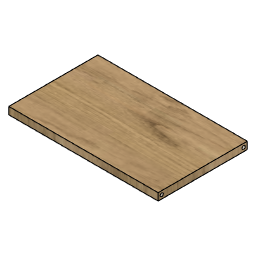
Project 02 (Autodesk Fusion 360 archive; units mm, degrees)
design "Base"
Autodesk Fusion 360 part; units mm, degrees
note: some values were not read from the file. Set by a fixed rule: which face or edge a step refers to.
sketch "Sketch1" plane through (0, 0, 0) normal (0, 1, 0) x (1, 0, 0)
  line L0 (0, 0) -> (310, 0)
  line L1 (310, 0) -> (310, -185)
  line L2 (310, -185) -> (0, -185)
  line L3 (0, -185) -> (0, 0)
  dimension "d1" = 310
  dimension "d2" = 185
  constraint horizontal L0
  constraint vertical L1
  constraint horizontal L2
  constraint vertical L3
  constraint coincident L0.start L3.end
  measures "d1" distance of L0.start L0.end
  measures "d2" distance of L0.start L2.end
extrude "Extrude1" add sketch "Sketch1" along normal blind 15
sketch "Sketch2" plane through (310, 0, 0) normal (1, 0, 0) x (0, 0, -1)
  line L0 (-185, 0) -> (0, 0)
  line L1 (0, 0) -> (0, 15)
  line L2 (0, 15) -> (-185, 15)
  line L3 (-185, 15) -> (-185, 0)
  circle A0 centre (-177.5, 7.5) radius 4
  circle A1 centre (-7.5, 7.5) radius 4
  line L4 (0, 0) -> (0, 7.5)
  constraint midpoint L1 L4.end
  constraint coincident L0.end L1.start
sketch "Sketch3" plane through (0, 0, 0) normal (-1, 0, 0) x (0, 0, 1)
  line L0 (0, 0) -> (185, 0)
  line L1 (185, 0) -> (185, 15)
  line L2 (185, 15) -> (0, 15)
  line L3 (0, 15) -> (0, 0)
  circle A0 centre (7.5, 7.5) radius 4
  dimension "d11" = 8
  measures "d11" diameter of A0
sketch "Sketch4" plane through (0, 0, 0) normal (-1, 0, 0) x (0, 0, 1)
  circle A0 centre (177.5, 7.5) radius 4
  line L0 (0, 0) -> (7.5, 0) construction
  line L1 (7.5, 0) -> (7.5, 7.5) construction
  line L2 (7.5, 7.5) -> (0, 7.5) construction
  line L3 (0, 7.5) -> (0, 0) construction
  circle A1 centre (7.5, 7.5) radius 4
  dimension "d75" = 7.5
  dimension "d76" = 7.5
  dimension "d77" = 8
  constraint horizontal L0
  constraint vertical L1
  constraint horizontal L2
  constraint vertical L3
  constraint coincident L0.start L3.end
  constraint coincident L1.end L2.start
  measures "d75" distance of L0.start L0.end
  measures "d76" distance of L0.start L2.end
  measures "d77" diameter of A1
extrude "Extrude2" cut sketch "Sketch2" against normal blind 3 contours A0 | A1
thread "Thread1" "ISO Metric profile 8.0 M8x1.25 6H" major diameter 8.17 minor diameter 6.7795 pitch 1.25 angle 60 resizes the face on face at (308, 7.3006, 3.505)
thread "Thread2" "ISO Metric profile 8.0 M8x1.25 6H" major diameter 8.17 minor diameter 6.7795 pitch 1.25 angle 60 resizes the face on face at (308, 10.3635, 180.2929)
sketch "Sketch5" plane through (0, 0, 0) normal (0, 0, -1) x (-1, 0, 0)
  line L0 (-310, 0) -> (0, 0)
  line L1 (0, 0) -> (0, 15)
  line L2 (0, 15) -> (-310, 15)
  line L3 (-310, 15) -> (-310, 0)
  circle A0 centre (-260, 7.5) radius 4
  line L4 (0, 7.5) -> (-50, 7.5)
  circle A1 centre (-50, 7.5) radius 4
  dimension "d21" = 50
  dimension "d22" = 8
  constraint midpoint L1 L4.start
  constraint perpendicular L1 L4
  constraint coincident L4.end A1.centre
  measures "d21" distance of L4.start L4.end
  measures "d22" diameter of A1
sketch "Sketch6" plane through (310, 0, 0) normal (1, 0, 0) x (0, 0, -1)
  circle A0 centre (-177.5, 7.5) radius 3.3898
  line L0 (-185, 0) -> (0, 0)
  line L1 (0, 0) -> (0, 15)
  line L2 (0, 15) -> (-185, 15)
  line L3 (-185, 15) -> (-185, 0)
  circle A1 centre (-7.5, 7.5) radius 4
  circle A2 centre (-7.5, 7.5) radius 3.3898
  dimension "d46" = 8
  measures "d46" diameter of A1
sketch "Sketch7" plane through (0, 0, 0) normal (0, 0, -1) x (-1, 0, 0)
  line L0 (-310, 0) -> (0, 0)
  line L1 (0, 0) -> (0, 15)
  line L2 (0, 15) -> (-310, 15)
  line L3 (-310, 15) -> (-310, 0)
  circle A0 centre (-260, 7.5) radius 4
  dimension "d48" = 8
  dimension "d52" = 0
  measures "d48" diameter of A0
extrude "Extrude16" cut sketch "Sketch7" against normal blind 30 contours A0
thread "Thread11" "ISO Metric profile 8.0 M8x1.25 6H" major diameter 8.17 minor diameter 6.7795 pitch 1.25 angle 60 resizes the face on face at (262.6467, 4.5009, 20)
delete_face "DeleteFace2" 1 faces at (258.4536, 10.5164, 20)
hole "Hole1" at (310, 7.5, 177.5) direction (-1, 0, 0) diameter 6.78 depth 30 tip angle 120
thread "Thread12" "ISO Metric profile 8.0 M8x1.25 6H"
hole "Hole2" at (310, 7.5, 7.5) direction (-1, 0, 0) diameter 6.78 depth 30 tip angle 120
thread "Thread13" "ISO Metric profile 8.0 M8x1.25 6H"
hole "Hole3" at (260, 7.5, 0) direction (0, 0, 1) diameter 6.78 depth 30 tip angle 120
thread "Thread14" "ISO Metric profile 8.0 M8x1.25 6H"
hole "Hole4" at (50, 7.5, 0) direction (0, 0, 1) diameter 6.78 depth 30 tip angle 120
thread "Thread15" "ISO Metric profile 8.0 M8x1.25 6H"
hole "Hole5" at (0, 7.5, 177.5) at (0, 7.5, 7.5) direction (1, 0, 0) diameter 6.78 depth 30 tip angle 120
thread "Thread16" "ISO Metric profile 8.0 M8x1.25 6H"

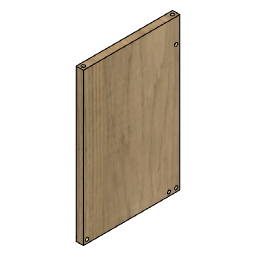
design "Left side"
Autodesk Fusion 360 part; units mm, degrees
sketch "Sketch1" plane through (0, 0, 0) normal (0, 1, 0) x (1, 0, 0)
  line L0 (0, 0) -> (15, 0)
  line L1 (15, 0) -> (15, -200)
  line L2 (15, -200) -> (0, -200)
  line L3 (0, -200) -> (0, 0)
  line L4 (325, -200) -> (340, -200)
  line L5 (340, -200) -> (340, 0)
  line L6 (340, 0) -> (325, 0)
  line L7 (325, 0) -> (325, -200)
  dimension "d1" = 15
  dimension "d2" = 200
  dimension "d3" = 310
  dimension "d4" = 15
  dimension "d5" = 200
  constraint horizontal L0
  constraint vertical L1
  constraint horizontal L2
  constraint vertical L3
  constraint coincident L0.start L3.end
  constraint horizontal L4
  constraint vertical L5
  constraint horizontal L6
  constraint vertical L7
  measures "d1" distance of L0.start L0.end
  measures "d2" distance of L0.start L2.end
  measures "d3" distance of L1.end L4.start
  measures "d4" distance of L4.start L4.end
  measures "d5" distance of L4.start L6.end
sketch "Sketch2" plane through (0, 0, 0) normal (0, 1, 0) x (1, 0, 0)
  line L0 (0, 0) -> (15, 0)
  line L1 (15, 0) -> (15, -200)
  line L2 (15, -200) -> (0, -200)
  line L3 (0, -200) -> (0, 0)
  dimension "d8" = 15
  dimension "d9" = 200
  constraint horizontal L0
  constraint vertical L1
  constraint horizontal L2
  constraint vertical L3
  constraint coincident L0.start L3.end
  measures "d8" distance of L0.start L0.end
  measures "d9" distance of L0.start L2.end
extrude "Extrude2" add sketch "Sketch2" along normal blind 315
sketch "Sketch3" plane through (0, 0, 0) normal (-1, 0, 0) x (0, 0, 1)
  line L0 (0, 0) -> (200, 0)
  line L1 (200, 0) -> (200, 315)
  line L2 (200, 315) -> (0, 315)
  line L3 (0, 315) -> (0, 0)
  circle A0 centre (7.5, 7.5) radius 4
  circle A1 centre (22.5, 7.5) radius 4
  circle A2 centre (192.5, 7.5) radius 4
  circle A3 centre (7.5, 265) radius 4
  dimension "d18" = 8
  dimension "d19" = 8
  dimension "d22" = 8
  dimension "d25" = 8
  measures "d18" diameter of A0
  measures "d19" diameter of A1
  measures "d22" diameter of A2
  measures "d25" diameter of A3
hole "Hole1" at (0, 7.5, 7.5) at (0, 7.5, 22.5) at (0, 265, 7.5) at (0, 7.5, 192.5) direction (1, 0, 0) diameter 6.78 depth 100 tip angle 120 countersink diameter 14.07 countersink angle 90
thread "Thread1" "ISO Metric profile 8.0 M8x1.25 6H"
sketch "Sketch4" plane through (0, 315, 0) normal (0, 1, 0) x (-1, 0, 0)
  line L0 (0, 200) -> (-15, 200)
  line L1 (-15, 200) -> (-15, 0)
  line L2 (-15, 0) -> (0, 0)
  line L3 (0, 0) -> (0, 200)
  circle A0 centre (-7.5, 192.5) radius 4
  circle A1 centre (-7.5, 7.5) radius 4
  dimension "d33" = 8
  dimension "d36" = 8
  measures "d33" diameter of A0
  measures "d36" diameter of A1
hole "Hole2" at (7.5, 315, 192.5) at (7.5, 315, 7.5) direction (0, -1, 0) diameter 6.78 depth 30 tip angle 120
thread "Thread2" "ISO Metric profile 8.0 M8x1.25 6H"

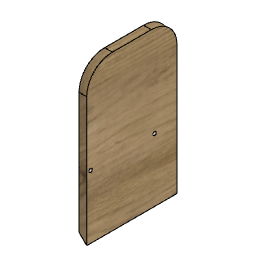
design "T-shape01"
Autodesk Fusion 360 part; units mm, degrees
sketch "Sketch1" plane through (0, 0, 0) normal (0, 1, 0) x (1, 0, 0)
  line L0 (0, 0) -> (21.213, 0)
  line L1 (0, -21.213) -> (0, -21.23)
  line L2 (-201.525, -201.525) -> (0, 0)
  line L3 (21.213, 0) -> (-190.919, -212.132)
  line L4 (-201.525, -201.525) -> (-190.919, -212.132)
  dimension "d1" = 21.213
  dimension "d2" = 21.23
  dimension "d5" = 300
  constraint coincident L0.start L2.end
  constraint horizontal L0
  constraint perpendicular L0 L1
  constraint parallel L2 L3
  constraint coincident L3 L1.start
  measures "d1" distance of L0.start L0.end
  measures "d2" distance of L0.start L1.end
  measures "d5" distance of L0.end L3.end
extrude "Extrude1" add sketch "Sketch1" along normal blind 175
sketch "Sketch2" plane through (10.6065, 0, 10.6065) normal (0.707107, 0, 0.707107) x (0, 1, 0)
  line L0 (0, 285.0001) -> (0, -14.9999)
  line L1 (0, -14.9999) -> (175, -14.9999)
  line L2 (175, -14.9999) -> (175, 285.0001)
  line L3 (175, 285.0001) -> (0, 285.0001)
  arc A0 (50, 285.0001) -> (0, 235.0001) centre (50, 235.0001) ccw
  arc A1 (175, 235.0001) -> (125, 285.0001) centre (125, 235.0001) ccw
  dimension "d8" = 250
  dimension "d9" = 50
  constraint coincident L3 A0.start
  measures "d8" distance of L0.end A0.end
  measures "d9" distance of A0.end A0.centre
extrude "Extrude2" cut sketch "Sketch2" against normal blind 60 contours L0 L3 A0
extrude "Extrude3" cut sketch "Sketch2" against normal blind 90 contours L2 L3 A1
sketch "Sketch3" plane through (0, 0, 0) normal (-0.707107, 0, -0.707107) x (0, -1, 0)
  arc A0 (-125.2749, 284.9994) -> (-175, 235.0001) centre (-125, 235.0001) ccw
  line L0 (-175, 235.0001) -> (-175, 0)
  line L1 (-175, 0) -> (0, 0)
  line L2 (0, 0) -> (0, 235.0001)
  arc A1 (0, 235.0001) -> (-49.7251, 284.9994) centre (-50, 235.0001) ccw
  line L3 (-49.7251, 284.9994) -> (-125.2749, 284.9994)
  line L4 (0, 0) -> (0, 107.5)
  line L5 (-175, 0) -> (-175, 107.5)
  line L6 (-175, 107.5) -> (-131.5, 107.5)
  line L7 (0, 107.5) -> (-7.5, 107.5)
  dimension "d15" = 107.5
  dimension "d16" = 107.5
  dimension "d17" = 43.5
  dimension "d18" = 7.5
  constraint coincident L1.end L2.start
  constraint perpendicular L1 L4
  constraint coincident L0.end L1.start
  constraint perpendicular L1 L5
  constraint perpendicular L0 L6
  constraint perpendicular L4 L7
  measures "d15" distance of L1.end L4.end
  measures "d16" distance of L0.end L5.end
  measures "d17" distance of L5.end L6.end
  measures "d18" distance of L4.end L7.end
hole "Hole1" at (-76.014, 131.5, 76.014) direction (0.707107, 0, 0.707107) diameter 6.78 depth 40 tip angle 120 countersink diameter 14.07 countersink angle 90
thread "Thread4" "ISO Metric profile 8.0 M8x1.25 6H"
thread "Thread1" "ISO Metric profile 8.0 M8x1.25 6H" major diameter 8.17 minor diameter 6.7795 pitch 1.25 angle 60 resizes the face on face at (-73.1387, 131.9215, 83.6462)
hole "Hole2" at (-76.014, 7.5, 76.014) direction (0.707107, 0, 0.707107) diameter 6.78 depth 40 tip angle 120 countersink diameter 14.07 countersink angle 90
thread "Thread3" "ISO Metric profile 8.0 M8x1.25 6H"
thread "Thread2" "ISO Metric profile 8.0 M8x1.25 6H" major diameter 8.17 minor diameter 6.7795 pitch 1.25 angle 60 resizes the face on face at (-67.9644, 10.8858, 83.8246)
sketch "Sketch4" plane through (0, 175, 0) normal (0, 1, 0) x (-1, 0, 0)
  line L0 (166.1702, 166.1702) -> (155.5637, 176.7767)
  line L1 (155.5637, 176.7767) -> (-21.213, 0)
  line L2 (-21.213, 0) -> (0, 0)
  line L3 (0, 0) -> (166.1702, 166.1702)
  circle A0 centre (17.6778, 28.2843) radius 4
  circle A1 centre (70.7108, 81.3173) radius 4
  circle A2 centre (113.1372, 123.7437) radius 4
  dimension "d26" = 75
  dimension "d27" = 60
  dimension "d28" = 8
  dimension "d29" = 8
  dimension "d30" = 8
  measures "d26" distance of A0.centre A1.centre
  measures "d27" distance of A1.centre A2.centre
  measures "d28" diameter of A0
  measures "d29" diameter of A1
  measures "d30" diameter of A2
hole "Hole3" at (-17.6778, 175, 28.2843) at (-70.7108, 175, 81.3173) at (-113.1372, 175, 123.7437) direction (0, -1, 0) diameter 6.78 depth 30 tip angle 120
thread "Thread5" "ISO Metric profile 8.0 M8x1.25 6H"
sketch "Sketch5" plane through (0, 0, 0) normal (0, 0, -1) x (1, 0, 0)
  line L0 (21.213, 0) -> (0, 0)
  line L1 (0, 0) -> (0, -175)
  line L2 (0, -175) -> (21.213, -175)
  line L3 (21.213, -175) -> (21.213, 0)
  circle A0 centre (10.6065, -24.08) radius 4
  circle A1 centre (10.6065, -170) radius 4
  dimension "d36" = 8
  dimension "d37" = 8
  measures "d36" diameter of A0
  measures "d37" diameter of A1
hole "Hole4" at (10.6065, 24.08, 0) at (10.6065, 170, 0) direction (0, 0, 1) diameter 6.78 depth 5 tip angle 120
thread "Thread6" "ISO Metric profile 8.0 M8x1.25 6H"
move_body "Move1" bodies 1 to x (0.707107, 0, -0.707107) y (0, 1, 0) z (0.707107, 0, 0.707107) at (-0.429, 0, 8.9644)

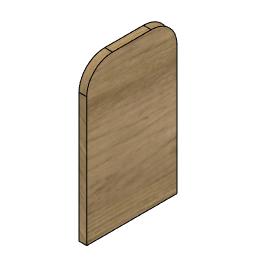
design "T-shape02"
Autodesk Fusion 360 part; units mm, degrees
sketch "Sketch1" plane through (0, 0, 0) normal (0, 0, 1) x (1, 0, 0)
sketch "Sketch2" plane through (0, 0, 0) normal (0, 0, 1) x (1, 0, 0)
  line L0 (0, 0) -> (9.9094, 0) construction
  line L1 (0, 0) -> (212.132, 212.132)
  line L2 (0, 0) -> (-10.6066, 10.6066)
  line L3 (-10.6066, 10.6066) -> (201.5254, 222.7386)
  line L4 (-10.6066, 10.6066) -> (289.3934, 10.6066) construction
  line L5 (212.132, 212.132) -> (201.5254, 222.7386)
  dimension "d2" = 300
  dimension "d3" = 15
  dimension "d4" = 45
  dimension "d5" = 300
  constraint horizontal L0
  constraint coincident L0.start L1.start
  constraint perpendicular L1 L2
  constraint horizontal L4
  constraint perpendicular L2 L3
  measures "d2" distance of L0.start L1.end
  measures "d3" distance of L0.start L2.end
  measures "d4" angle of L3 L4
  measures "d5" distance of L2.end L3.end
extrude "Extrude1" add sketch "Sketch2" along normal blind 175
sketch "Sketch3" plane through (-10.6066, 10.6066, 0) normal (-0.707107, 0.707107, 0) x (0, 0, 1)
  line L0 (0, 300) -> (0, 0)
  line L1 (0, 0) -> (175, 0)
  line L2 (175, 0) -> (175, 300)
  line L3 (175, 300) -> (0, 300)
  arc A0 (50, 300) -> (0, 250) centre (50, 250) ccw
  arc A1 (175, 250) -> (125, 300) centre (125, 250) ccw
  dimension "d8" = 100
  constraint tangent L2 A1
  constraint coincident L0 A0.end
  constraint coincident L3 A1.end
  measures "d8" diameter of A0
extrude "Extrude2" cut sketch "Sketch3" against normal blind 175 contours L0 L3 A0
extrude "Extrude3" cut sketch "Sketch3" against normal blind 175 contours L2 L3 A1
sketch "Sketch4" plane through (0, 0, 0) normal (-0.707107, -0.707107, 0) x (0, 0, 1)
  line L0 (0, 15) -> (0, 0)
  line L1 (0, 0) -> (175, 0)
  line L2 (175, 0) -> (175, 15)
  line L3 (175, 15) -> (0, 15)
sketch "Sketch7" plane through (0, 0, 0) normal (0, 0, 1) x (1, 0, 0)
  circle A0 centre (53.033, 63.6396) radius 4
  dimension "d27" = 8
  measures "d27" diameter of A0
extrude "Extrude4" cut sketch "Sketch7" along normal blind 30
sketch "Sketch8" plane through (0, 0, 0) normal (-0.707107, -0.707107, 0) x (0, 0, 1)
  line L0 (0, 15) -> (0, 0)
  line L1 (0, 0) -> (175, 0)
  line L2 (175, 0) -> (175, 15)
  line L3 (175, 15) -> (0, 15)
  circle A0 centre (167.5, 7.5) radius 4
  circle A1 centre (43.5, 7.5) radius 4
  dimension "d32" = 8
  dimension "d33" = 124
  dimension "d34" = 8
  measures "d32" diameter of A0
  measures "d33" distance of A0.centre A1.centre
  measures "d34" diameter of A1
hole "Hole2" at (-5.3033, 5.3033, 43.5) at (-5.3033, 5.3033, 167.5) direction (0.707107, 0.707107, 0) diameter 6.78 depth 30 tip angle 118
thread "Thread3" "ISO Metric profile 8.0 M8x1.25 6H"
move_body "MoveFace1" bodies 1 to x (0.707107, 0.707107, 0) y (-0.707107, 0.707107, 0) z (0, 0, 1) at (92.7817, -26.0051, 0)
extrude "Extrude5" add 1 faces at (86.1181, 54.2391, 30) along direction (0, 0, -1) blind 25
extrude "Extrude6" add 1 faces at (86.1181, 54.2391, 5) along direction (0, 0, -1) blind 5
sketch "Sketch9" plane through (0, 0, 0) normal (0, 0, -1) x (-1, 0, 0)
  line L0 (-77.7817, 223.9949) -> (-92.7817, 223.9949)
  line L1 (-92.7817, 223.9949) -> (-92.7817, -26.0051)
  line L2 (-92.7817, -26.0051) -> (-77.7817, -26.0051)
  line L3 (-77.7817, -26.0051) -> (-77.7817, 223.9949)
  circle A0 centre (-85.2817, 56.4949) radius 4
  dimension "d43" = 8
  measures "d43" diameter of A0
hole "Hole3" at (85.2817, 56.4949, 0) direction (0, 0, 1) diameter 6.78 depth 30 tip angle 118
thread "Thread4" "ISO Metric profile 8.0 M8x1.25 6H"

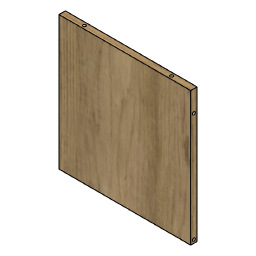
design "Back side"
Autodesk Fusion 360 part; units mm, degrees
sketch "Sketch1" plane through (0, 0, 0) normal (0, 1, 0) x (1, 0, 0)
  line L0 (0, 0) -> (310, 0)
  line L1 (310, 0) -> (310, -15)
  line L2 (310, -15) -> (0, -15)
  line L3 (0, -15) -> (0, 0)
  dimension "d1" = 310
  dimension "d2" = 15
  constraint horizontal L0
  constraint vertical L1
  constraint horizontal L2
  constraint vertical L3
  constraint coincident L0.start L3.end
  measures "d1" distance of L0.start L0.end
  measures "d2" distance of L0.start L2.end
extrude "Extrude1" add sketch "Sketch1" along normal blind 315
sketch "Sketch2" plane through (310, 0, 0) normal (1, 0, 0) x (0, 0, -1)
  line L0 (-15, 0) -> (0, 0)
  line L1 (0, 0) -> (0, 315)
  line L2 (0, 315) -> (-15, 315)
  line L3 (-15, 315) -> (-15, 0)
  line L4 (0, 0) -> (-7.5, 0) construction
  line L5 (-7.5, 0) -> (-7.5, 7.5) construction
  line L6 (-7.5, 7.5) -> (0, 7.5) construction
  line L7 (0, 7.5) -> (0, 0) construction
  circle A0 centre (-7.5, 7.5) radius 4
  line L8 (-15, 315) -> (-7.5, 315) construction
  line L9 (-7.5, 315) -> (-7.5, 265) construction
  line L10 (-7.5, 265) -> (-15, 265) construction
  line L11 (-15, 265) -> (-15, 315) construction
  circle A1 centre (-7.5, 265) radius 4
  dimension "d5" = 7.5
  dimension "d6" = 7.5
  dimension "d7" = 8
  dimension "d8" = 50
  dimension "d9" = 8
  constraint horizontal L4
  constraint vertical L5
  constraint horizontal L6
  constraint vertical L7
  constraint coincident L0.end L1.start
  constraint coincident L5.end L6.start
  constraint horizontal L8
  constraint vertical L9
  constraint horizontal L10
  constraint vertical L11
  constraint coincident L2.end L3.start
  constraint coincident L9.end L10.start
  measures "d5" distance of L0.end L4.end
  measures "d6" distance of L0.end L6.end
  measures "d7" diameter of A0
  measures "d8" distance of L2.end L10.end
  measures "d9" diameter of A1
sketch "Sketch3" plane through (310, 0, 0) normal (1, 0, 0) x (0, 1, 0)
sketch "Sketch4" plane through (0, 315, 0) normal (0, 1, 0) x (-1, 0, 0)
  line L0 (0, 15) -> (-310, 15)
  line L1 (-310, 15) -> (-310, 0)
  line L2 (-310, 0) -> (0, 0)
  line L3 (0, 0) -> (0, 15)
  line L4 (0, 0) -> (-60, 0) construction
  line L5 (-60, 0) -> (-52.5, 0) construction
  line L6 (-52.5, 0) -> (-52.5, 7.5) construction
  line L7 (-52.5, 7.5) -> (-60, 7.5) construction
  line L8 (-60, 7.5) -> (-60, 0) construction
  circle A0 centre (-52.5, 7.5) radius 4
  line L9 (-310, 0) -> (-300, 0) construction
  line L10 (-310, 0) -> (-250, 0) construction
  line L11 (-250, 0) -> (-257.5, 0) construction
  line L12 (-257.5, 0) -> (-257.5, 7.5) construction
  line L13 (-257.5, 7.5) -> (-250, 7.5) construction
  line L14 (-250, 7.5) -> (-250, 0) construction
  circle A1 centre (-257.5, 7.5) radius 4
  dimension "d10" = 60
  dimension "d11" = 7.5
  dimension "d12" = 7.5
  dimension "d13" = 8
  dimension "d14" = 60
  dimension "d15" = 7.5
  dimension "d16" = 7.5
  dimension "d17" = 8
  constraint coincident L2.end L3.start
  constraint perpendicular L3 L4
  constraint horizontal L5
  constraint vertical L6
  constraint horizontal L7
  constraint vertical L8
  constraint coincident L6.end L7.start
  constraint coincident L1.end L2.start
  constraint coincident L2 L9.end
  constraint perpendicular L1 L9
  constraint perpendicular L1 L10
  constraint horizontal L11
  constraint vertical L12
  constraint horizontal L13
  constraint vertical L14
  constraint coincident L12.end L13.start
  measures "d10" distance of L2.end L4.end
  measures "d11" distance of L4.end L5.end
  measures "d12" distance of L4.end L7.end
  measures "d13" diameter of A0
  measures "d14" distance of L1.end L10.end
  measures "d15" distance of L10.end L11.end
  measures "d16" distance of L10.end L13.end
  measures "d17" diameter of A1
sketch "Sketch5" plane through (0, 0, 0) normal (-1, 0, 0) x (0, 0, 1)
  line L0 (0, 0) -> (15, 0)
  line L1 (15, 0) -> (15, 315)
  line L2 (15, 315) -> (0, 315)
  line L3 (0, 315) -> (0, 0)
  line L4 (0, 0) -> (7.5, 0) construction
  line L5 (7.5, 0) -> (7.5, 7.5) construction
  line L6 (7.5, 7.5) -> (0, 7.5) construction
  line L7 (0, 7.5) -> (0, 0) construction
  circle A0 centre (7.5, 7.5) radius 4
  line L8 (0, 315) -> (7.5, 315) construction
  line L9 (7.5, 315) -> (7.5, 265) construction
  line L10 (7.5, 265) -> (0, 265) construction
  line L11 (0, 265) -> (0, 315) construction
  circle A1 centre (7.5, 265) radius 4
  dimension "d18" = 7.5
  dimension "d19" = 7.5
  dimension "d20" = 8
  dimension "d21" = 50
  dimension "d22" = 8
  constraint horizontal L4
  constraint vertical L5
  constraint horizontal L6
  constraint vertical L7
  constraint coincident L0.start L3.end
  constraint coincident L5.end L6.start
  constraint horizontal L8
  constraint vertical L9
  constraint horizontal L10
  constraint vertical L11
  constraint coincident L2.end L3.start
  constraint coincident L9.end L10.start
  measures "d18" distance of L0.start L4.end
  measures "d19" distance of L0.start L6.end
  measures "d20" diameter of A0
  measures "d21" distance of L2.end L10.end
  measures "d22" diameter of A1
hole "Hole2" at (0, 265, 7.5) at (0, 7.5, 7.5) direction (1, 0, 0) diameter 6.78 depth 30 tip angle 120
thread "Thread1" "ISO Metric profile 8.0 M8x1.25 6H"
hole "Hole3" at (52.5, 315, 7.5) at (257.5, 315, 7.5) direction (0, -1, 0) diameter 6.78 depth 30 tip angle 120
thread "Thread2" "ISO Metric profile 8.0 M8x1.25 6H"
hole "Hole4" at (310, 265, 7.5) at (310, 7.5, 7.5) direction (-1, 0, 0) diameter 6.78 depth 30 tip angle 120
thread "Thread3" "ISO Metric profile 8.0 M8x1.25 6H"

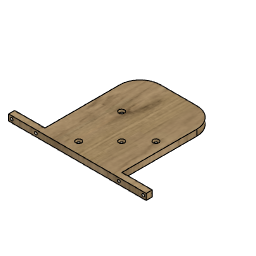
design "Upper back side"
Autodesk Fusion 360 part; units mm, degrees
sketch "Sketch1" plane through (0, 0, 0) normal (0, 0, 1) x (1, 0, 0)
  line L0 (0, 0) -> (340, 0)
  line L1 (340, 0) -> (0, 0)
  line L2 (0, 0) -> (0, 250)
  line L3 (0, 250) -> (340, 250)
  line L4 (340, 250) -> (340, 0)
  line L5 (0, 0) -> (0, 15)
  line L6 (0, 15) -> (75, 15)
  line L7 (340, 0) -> (340, 15)
  line L8 (340, 15) -> (265, 15)
  line L9 (75, 15) -> (75, 250)
  line L10 (265, 15) -> (265, 250)
  dimension "d1" = 340
  dimension "d2" = 340
  dimension "d3" = 250
  dimension "d4" = 15
  dimension "d5" = 75
  dimension "d6" = 15
  dimension "d7" = 75
  constraint coincident L0.start L1.end
  constraint horizontal L0
  constraint horizontal L1
  constraint vertical L2
  constraint horizontal L3
  constraint vertical L4
  constraint parallel L2 L5
  constraint perpendicular L5 L6
  constraint perpendicular L0 L7
  constraint perpendicular L4 L8
  constraint coincident L3 L9.end
  constraint perpendicular L3 L9
  constraint coincident L3 L10.end
  constraint perpendicular L3 L10
  measures "d1" distance of L0.start L0.end
  measures "d2" distance of L0.end L0.start
  measures "d3" distance of L0.start L2.end
  measures "d4" distance of L0.start L5.end
  measures "d5" distance of L5.end L6.end
  measures "d6" distance of L0.end L7.end
  measures "d7" distance of L7.end L8.end
extrude "Extrude1" add sketch "Sketch1" against normal blind 15 contours L0 L1 L2 L3 L4 L5 L6 L7 L8 L9 L10
fillet "Fillet1" radius 50 1 edges at (265, 250, -7.5)
fillet "Fillet2" radius 50 1 edges at (75, 250, -7.5)
sketch "Sketch2" plane through (0, 0, 0) normal (0, 0, 1) x (1, 0, 0)
  line L0 (0, 15) -> (131.607, 15)
  line L1 (131.607, 15) -> (250.8741, 134.2671)
  line L2 (131.607, 15) -> (144.8914, 28.2844)
  line L3 (340, 0) -> (0, 0)
  line L4 (144.8914, 28.2844) -> (197.9244, 81.3174)
  circle A0 centre (197.9244, 81.3174) radius 4
  circle A1 centre (144.8914, 28.2844) radius 4
  line L5 (197.9244, 81.3174) -> (240.3508, 123.7438)
  line L6 (197.9244, 81.3174) -> (134.2848, 144.957)
  circle A2 centre (134.2848, 144.957) radius 4
  circle A3 centre (240.3508, 123.7438) radius 4
  point P0 (0, 15)
  dimension "d14" = 131.607
  dimension "d15" = 135
  dimension "d16" = 18.787
  dimension "d17" = 28.2844
  dimension "d18" = 75
  dimension "d19" = 8
  dimension "d20" = 8
  dimension "d21" = 60
  dimension "d22" = 90
  dimension "d23" = 8
  dimension "d24" = 8
  constraint coincident P0 L0.start
  constraint parallel L1 L2
  constraint parallel L1 L4
  constraint coincident L4.end A0.centre
  constraint coincident L2.end L4.start
  constraint parallel L1 L5
  constraint perpendicular L4 L6
  constraint coincident L6.end A2.centre
  constraint coincident L5.end A3.centre
  measures "d14" distance of P0 L0.end
  measures "d15" angle of L0 L1
  measures "d16" distance of L0.end L2.end
  measures "d17" distance of L2.end L3
  measures "d18" distance of L2.end L4.end
  measures "d19" diameter of A0
  measures "d20" diameter of A1
  measures "d21" distance of L4.end L5.end
  measures "d22" distance of L4.end L6.end
  measures "d23" diameter of A2
  measures "d24" diameter of A3
hole "Hole1" at (134.2848, 144.957, 0) at (197.9244, 81.3174, 0) at (144.8914, 28.2844, 0) at (240.3508, 123.7438, 0) direction (0, 0, -1) diameter 6.78 depth 30 tip angle 118 countersink diameter 14.07 countersink angle 90
thread "Thread1" "ISO Metric profile 8.0 M8x1.25 6H"
sketch "Sketch3" plane through (0, 15, 0) normal (0, 1, 0) x (-1, 0, 0)
  line L0 (0, 0) -> (-75, 0)
  line L1 (-75, 0) -> (-75, -15)
  line L2 (-75, -15) -> (0, -15)
  line L3 (0, -15) -> (0, 0)
  line L4 (0, 0) -> (-7.5, 0)
  line L5 (-7.5, 0) -> (-7.5, -7.5)
  line L6 (-75, 0) -> (-75, -7.5)
  line L7 (-75, -7.5) -> (-67.5, -7.5)
  line L8 (-265, 0) -> (-265, -7.5)
  line L9 (-265, -7.5) -> (-272.5, -7.5)
  line L10 (-340, 0) -> (-340, -7.5)
  line L11 (-340, -7.5) -> (-332.5, -7.5)
  point P0 (-265, 0)
  point P1 (-340, 0)
  dimension "d30" = 7.5
  dimension "d31" = 7.5
  dimension "d32" = 7.5
  dimension "d33" = 7.5
  dimension "d34" = 7.5
  dimension "d35" = 7.5
  dimension "d36" = 7.5
  dimension "d37" = 7.5
  constraint coincident L0.start L3.end
  constraint perpendicular L3 L4
  constraint perpendicular L0 L5
  constraint coincident L0.end L1.start
  constraint perpendicular L0 L6
  constraint perpendicular L6 L7
  constraint coincident P0 L8.start
  constraint perpendicular L8 L9
  constraint coincident P1 L10.start
  constraint perpendicular L10 L11
  measures "d30" distance of L0.start L4.end
  measures "d31" distance of L4.end L5.end
  measures "d32" distance of L0.end L6.end
  measures "d33" distance of L6.end L7.end
  measures "d34" distance of P0 L8.end
  measures "d35" distance of L8.end L9.end
  measures "d36" distance of P1 L10.end
  measures "d37" distance of L10.end L11.end
hole "Hole2" at (272.5, 15, -7.5) at (332.5, 15, -7.5) at (67.5, 15, -7.5) at (7.5, 15, -7.5) direction (0, -1, 0) diameter 6.78 depth 30 tip angle 118 countersink diameter 14.07 countersink angle 90
thread "Thread2" "ISO Metric profile 8.0 M8x1.25 6H"

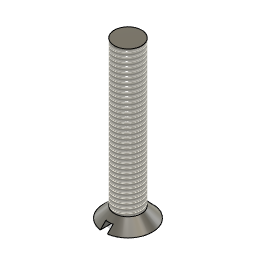
design "Flat Screw M8x1.25 45mm"
Autodesk Fusion 360 part; units mm, degrees
sketch "Sketch1" plane through (0, 0, 0) normal (0, 0, 1) x (1, 0, 0)
  line L0 (7.035, 0) -> (0, 0)
  line L1 (0, 0) -> (-7.035, 0)
  line L2 (-7.035, 0) -> (0, 7.035)
  line L3 (0, 7.035) -> (7.035, 0)
  line L4 (0, 0) -> (4, 0)
  line L5 (4, 0) -> (-4, 0)
  line L6 (-4, 0) -> (-4, 45)
  line L7 (-4, 45) -> (4, 45)
  line L8 (4, 45) -> (4, 0)
  line L9 (0, 45) -> (0, 0)
  dimension "d1" = 7.035
  dimension "d2" = 7.035
  dimension "d3" = 45
  dimension "d4" = 4
  dimension "d5" = 8
  dimension "d6" = 45
  constraint horizontal L0
  constraint coincident L0.end L1.start
  constraint parallel L0 L1
  constraint perpendicular L2 L3
  constraint parallel L0 L4
  constraint horizontal L5
  constraint vertical L6
  constraint horizontal L7
  constraint vertical L8
  constraint midpoint L7 L9.start
  measures "d1" distance of L0.start L0.end
  measures "d2" distance of L0.end L1.end
  measures "d3" angle of L1 L2
  measures "d4" distance of L0.end L4.end
  measures "d5" distance of L4.end L5.end
  measures "d6" distance of L4.end L7.end
revolve "Revolve1" add sketch "Sketch1" angle 360 about axis through (0, 45, 0) along (0, -1, 0) contours L1 L2 L5 L6 L9 | L2 L6 L7 L9 | L1 L2 L6
thread "Thread1" "ISO Metric profile 8.0 M8x1.25 6g" major diameter 7.866 minor diameter 6.4455 pitch 1.25 angle 60 resizes the face on face at (-3.995, 17.0233, 0.1994)
sketch "Sketch2" plane through (0, 0, 0) normal (0, 0, 1) x (1, 0, 0)
  line L0 (-1.03, 0) -> (1.03, 0)
  line L1 (1.03, 0) -> (1.03, 1.6)
  line L2 (1.03, 1.6) -> (-1.03, 1.6)
  line L3 (-1.03, 1.6) -> (-1.03, 0)
  constraint horizontal L0
  constraint vertical L1
  constraint horizontal L2
  constraint vertical L3
  constraint coincident origin L0
extrude "Extrude1" cut sketch "Sketch2" along normal blind 8 and the other way blind 7.5
equation "d1 = ( 14.07 / 2 ) * 1 mm"

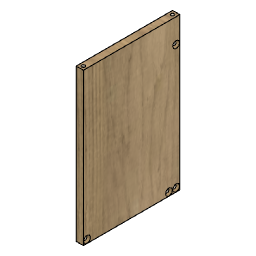
design "Right side"
Autodesk Fusion 360 part; units mm, degrees
sketch "Sketch1" plane through (0, 0, 0) normal (0, 1, 0) x (1, 0, 0)
  line L0 (325, 0) -> (340, 0)
  line L1 (340, 0) -> (340, -200)
  line L2 (340, -200) -> (325, -200)
  line L3 (325, -200) -> (325, 0)
  dimension "d4" = 15
  dimension "d5" = 200
  constraint horizontal L0
  constraint vertical L1
  constraint horizontal L2
  constraint vertical L3
  measures "d4" distance of L0.start L0.end
  measures "d5" distance of L0.start L2.end
extrude "Extrude1" add sketch "Sketch1" along normal blind 315
sketch "Sketch2" plane through (340, 0, 0) normal (1, 0, 0) x (0, 0, -1)
  line L0 (-200, 0) -> (0, 0)
  line L1 (0, 0) -> (0, 315)
  line L2 (0, 315) -> (-200, 315)
  line L3 (-200, 315) -> (-200, 0)
  circle A0 centre (-7.5, 265) radius 4
  circle A1 centre (-192.5, 7.5) radius 4
  circle A2 centre (-7.5, 7.5) radius 4
  circle A3 centre (-22.5, 7.5) radius 4
  dimension "d10" = 8
  dimension "d13" = 8
  dimension "d20" = 8
  dimension "d21" = 8
  measures "d10" diameter of A0
  measures "d13" diameter of A1
  measures "d20" diameter of A2
  measures "d21" diameter of A3
hole "Hole1" at (340, 265, 7.5) at (340, 7.5, 7.5) at (340, 7.5, 22.5) at (340, 7.5, 192.5) direction (-1, 0, 0) diameter 6.78 depth 100 tip angle 120 countersink diameter 14.07 countersink angle 90
thread "Thread1" "ISO Metric profile 8.0 M8x1.25 6H"
sketch "Sketch3" plane through (0, 315, 0) normal (0, 1, 0) x (-1, 0, 0)
  line L0 (-325, 200) -> (-340, 200)
  line L1 (-340, 200) -> (-340, 0)
  line L2 (-340, 0) -> (-325, 0)
  line L3 (-325, 0) -> (-325, 200)
  circle A0 centre (-332.5, 192.5) radius 4
  circle A1 centre (-332.5, 7.5) radius 4
  dimension "d29" = 8
  dimension "d32" = 8
  measures "d29" diameter of A0
  measures "d32" diameter of A1
hole "Hole2" at (332.5, 315, 7.5) at (332.5, 315, 192.5) direction (0, -1, 0) diameter 6.78 depth 30 tip angle 120
thread "Thread2" "ISO Metric profile 8.0 M8x1.25 6H"

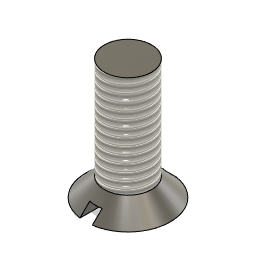
design "Flat Screw M8x1.25 20mm"
Autodesk Fusion 360 part; units mm, degrees
sketch "Sketch1" plane through (0, 0, 0) normal (0, 0, 1) x (1, 0, 0)
  line L0 (0, 0) -> (7.035, 0)
  line L1 (7.035, 0) -> (-7.035, 0)
  line L2 (-7.035, 0) -> (0, 7.035)
  line L3 (-7.035, 0) -> (2.914, 0) construction
  line L4 (0, 7.035) -> (7.035, 0)
  line L5 (0, 0) -> (4, 0) construction
  line L6 (4, 0) -> (-4, 0)
  line L7 (-4, 0) -> (-4, 20)
  line L8 (-4, 20) -> (4, 20)
  line L9 (4, 20) -> (4, 0)
  line L10 (0, 0) -> (1.03, 0) construction
  line L11 (1.03, 0) -> (1.03, 1.6) construction
  line L12 (1.03, 0) -> (-1.03, 0)
  line L13 (-1.03, 0) -> (-1.03, 1.6)
  line L14 (-1.03, 1.6) -> (1.03, 1.6)
  line L15 (1.03, 1.6) -> (1.03, 0)
  line L16 (0, 0) -> (0, 20)
  dimension "d1" = 7.035
  dimension "d2" = 14.07
  dimension "d3" = 45
  dimension "d4" = 4
  dimension "d5" = 8
  dimension "d6" = 20
  dimension "d7" = 1.03
  dimension "d8" = 1.6
  dimension "d9" = 2.06
  dimension "d10" = 1.6
  constraint coincident L0.start L5.start
  constraint horizontal L0
  constraint parallel L0 L1
  constraint horizontal L3
  constraint perpendicular L2 L4
  constraint parallel L1 L5
  constraint horizontal L6
  constraint vertical L7
  constraint horizontal L8
  constraint vertical L9
  constraint parallel L3 L10
  constraint perpendicular L5 L11
  constraint horizontal L12
  constraint vertical L13
  constraint horizontal L14
  constraint vertical L15
  constraint midpoint L8 L16.end
  measures "d1" distance of L0.start L0.end
  measures "d2" distance of L0.end L1.end
  measures "d3" angle of L2 L3
  measures "d4" distance of L0.start L5.end
  measures "d5" distance of L5.end L6.end
  measures "d6" distance of L5.end L8.end
  measures "d7" distance of L0.start L10.end
  measures "d8" distance of L10.end L11.end
  measures "d9" distance of L10.end L12.end
  measures "d10" distance of L10.end L11.end
revolve "Revolve1" add sketch "Sketch1" angle 360 about axis through (0, 0, 0) along (0, 1, 0) contours L1 L6 L12 L13 L14 L16 | L1 L2 L6 L7 L13 L14 L16 | L1 L2 L7 | L2 L7 L8 L16
extrude "Extrude1" cut sketch "Sketch1" along normal blind 10 and the other way blind 9 contours L0 L1 L6 L12 L14 L15 L16 | L1 L6 L12 L13 L14 L16
thread "Thread1" "ISO Metric profile 8.0 M8x1.25 6g" major diameter 7.866 minor diameter 6.4455 pitch 1.25 angle 60 resizes the face on face at (-3.995, 8.69, -0.1994)
equation "d2 = ( 7.035 * 2 ) * 1 mm"

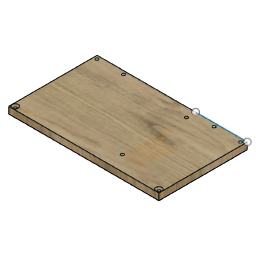
design "Upper Base"
Autodesk Fusion 360 part; units mm, degrees
sketch "Sketch1" plane through (0, 0, 0) normal (0, 1, 0) x (1, 0, 0)
  line L0 (0, 0) -> (340, 0)
  line L1 (340, 0) -> (340, -200)
  line L2 (340, -200) -> (0, -200)
  line L3 (0, -200) -> (0, 0)
  dimension "d1" = 340
  dimension "d2" = 200
  constraint horizontal L0
  constraint vertical L1
  constraint horizontal L2
  constraint vertical L3
  constraint coincident L0.start L3.end
  measures "d1" distance of L0.start L0.end
  measures "d2" distance of L0.start L2.end
extrude "Extrude1" add sketch "Sketch1" along normal blind 15
sketch "Sketch2" plane through (0, 15, 0) normal (0, 1, 0) x (-1, 0, 0)
  line L0 (0, 200) -> (-340, 200)
  line L1 (-340, 200) -> (-340, 0)
  line L2 (-340, 0) -> (0, 0)
  line L3 (0, 0) -> (0, 200)
sketch "Sketch3" plane through (0, 15, 0) normal (0, 1, 0) x (-1, 0, 0)
  circle A0 centre (-332.5, 192.5) radius 4
  line L0 (-340, 0) -> (-340, 7.5)
  circle A1 centre (-332.5, 7.5) radius 4
  line L1 (0, 200) -> (0, 192.5)
  circle A2 centre (-10.5, 192.5) radius 4
  dimension "d7" = 8
  dimension "d8" = 7.5
  dimension "d9" = 7.5
  dimension "d10" = 8
  dimension "d11" = 7.5
  dimension "d12" = 8
  constraint vertical L0
  constraint vertical L1
  measures "d7" diameter of A0
  measures "d8" distance of L0.start L0.end
  measures "d9" distance of L0.end A1.centre
  measures "d10" diameter of A1
  measures "d11" distance of L1.start L1.end
  measures "d12" diameter of A2
sketch "Sketch4" plane through (0, 15, 0) normal (0, 1, 0) x (-1, 0, 0)
  line L0 (0, 0) -> (0, 7.5)
  line L1 (0, 7.5) -> (-7.5, 7.5)
  circle A0 centre (-7.5, 7.5) radius 4
  line L2 (-340, 0) -> (-272.5, 0)
  line L3 (-272.5, 0) -> (-272.5, 7.5)
  circle A1 centre (-272.5, 7.5) radius 4
  line L4 (-340, 0) -> (-223, 0)
  line L5 (-223, 0) -> (-223, 20)
  circle A2 centre (-223, 20) radius 4
  line L6 (0, 0) -> (-67.5, 0)
  line L7 (-67.5, 0) -> (-67.5, 7.5)
  circle A3 centre (-67.5, 7.5) radius 4
  line L8 (-340, 200) -> (-223.907, 200)
  line L9 (-223.907, 200) -> (-223.907, 165.92)
  circle A4 centre (-223.907, 165.92) radius 4
  dimension "d13" = 7.5
  dimension "d14" = 7.5
  dimension "d15" = 8
  dimension "d16" = 67.5
  dimension "d17" = 7.5
  dimension "d18" = 8
  dimension "d19" = 117
  dimension "d20" = 20
  dimension "d21" = 8
  dimension "d22" = 67.5
  dimension "d23" = 7.5
  dimension "d24" = 8
  dimension "d25" = 116.093
  dimension "d26" = 34.08
  dimension "d27" = 8
  constraint coincident L0.start L6.start
  constraint vertical L0
  constraint perpendicular L0 L1
  constraint coincident L1.end A0.centre
  constraint horizontal L2
  constraint perpendicular L2 L3
  constraint coincident L3.end A1.centre
  constraint parallel L2 L4
  constraint perpendicular L2 L5
  constraint coincident L5.end A2.centre
  constraint perpendicular L0 L6
  constraint perpendicular L6 L7
  constraint coincident L7.end A3.centre
  constraint horizontal L8
  constraint perpendicular L8 L9
  constraint coincident L9.end A4.centre
  measures "d13" distance of L0.start L0.end
  measures "d14" distance of L0.end L1.end
  measures "d15" diameter of A0
  measures "d16" distance of L2.start L2.end
  measures "d17" distance of L2.end L3.end
  measures "d18" diameter of A1
  measures "d19" distance of L2.start L4.end
  measures "d20" distance of L4.end L5.end
  measures "d21" diameter of A2
  measures "d22" distance of L0.start L6.end
  measures "d23" distance of L6.end L7.end
  measures "d24" diameter of A3
  measures "d25" distance of L8.start L8.end
  measures "d26" distance of L8.end L9.end
  measures "d27" diameter of A4
extrude "Extrude2" cut sketch "Sketch4" sketch "Sketch3" against normal blind 130 of sketch 2
thread "Thread1" "ISO Metric profile 8.0 M8x1.25 6H" major diameter 8.17 minor diameter 6.7795 pitch 1.25 angle 60 resizes the face on face at (14.2588, 5, 193.8681)
thread "Thread2" "ISO Metric profile 8.0 M8x1.25 6H" major diameter 8.17 minor diameter 6.7795 pitch 1.25 angle 60 resizes the face on face at (221.2603, 10, 162.9209)
thread "Thread3" "ISO Metric profile 8.0 M8x1.25 6H" major diameter 8.17 minor diameter 6.7795 pitch 1.25 angle 60 resizes the face on face at (328.8141, 5, 194.0537)
thread "Thread4" "ISO Metric profile 8.0 M8x1.25 6H" major diameter 8.17 minor diameter 6.7795 pitch 1.25 angle 60 resizes the face on face at (3.5199, 5, 7.1017)
thread "Thread5" "ISO Metric profile 8.0 M8x1.25 6H" major diameter 8.17 minor diameter 6.7795 pitch 1.25 angle 60 resizes the face on face at (63.5199, 5, 7.1017)
thread "Thread6" "ISO Metric profile 8.0 M8x1.25 6H" major diameter 8.17 minor diameter 6.7795 pitch 1.25 angle 60 resizes the face on face at (220.8298, 10, 16.6399)
thread "Thread7" "ISO Metric profile 8.0 M8x1.25 6H" major diameter 8.17 minor diameter 6.7795 pitch 1.25 angle 60 resizes the face on face at (275.2929, 10, 4.6365)
thread "Thread8" "ISO Metric profile 8.0 M8x1.25 6H" major diameter 8.17 minor diameter 6.7795 pitch 1.25 angle 60 resizes the face on face at (335.1467, 5, 4.5009)
sketch "Sketch5" plane through (0, 15, 0) normal (0, 1, 0) x (-1, 0, 0)
delete_face "DeleteFace1" 1 faces at (227.1919, 5, 165.0836)
delete_face "DeleteFace2" 1 faces at (330.9536, 5, 195.5164)
delete_face "DeleteFace3" 1 faces at (222.9155, 10, 23.3887)
delete_face "DeleteFace4" 1 faces at (13.7849, 5, 191.6636)
sketch "Sketch6" plane through (0, 15, 0) normal (0, 1, 0) x (-1, 0, 0)
  circle A0 centre (-272.5, 7.5) radius 3.3898
  circle A1 centre (-7.5, 7.5) radius 3.3898
  circle A2 centre (-67.5, 7.5) radius 3.3898
  circle A3 centre (-332.5, 7.5) radius 3.3898
  line L0 (0, 200) -> (-340, 200)
  line L1 (-340, 200) -> (-340, 0)
  line L2 (-340, 0) -> (0, 0)
  line L3 (0, 0) -> (0, 200)
  line L4 (0, 200) -> (0, 192.5)
  line L5 (0, 192.5) -> (-7.5, 192.5)
  line L6 (-340, 200) -> (-340, 192.5)
  line L7 (-340, 192.5) -> (-332.5, 192.5)
  dimension "d30" = 7.5
  dimension "d31" = 7.5
  dimension "d32" = 7.5
  dimension "d33" = 7.5
  constraint coincident L0.start L3.end
  constraint perpendicular L0 L4
  constraint perpendicular L4 L5
  constraint coincident L0.end L1.start
  constraint perpendicular L0 L6
  constraint perpendicular L6 L7
  measures "d30" distance of L0.start L4.end
  measures "d31" distance of L4.end L5.end
  measures "d32" distance of L0.end L6.end
  measures "d33" distance of L6.end L7.end
sketch "Sketch7" plane through (0, 15, 0) normal (0, 1, 0) x (-1, 0, 0)
  circle A0 centre (-7.5, 192.5) radius 4
  dimension "d34" = 8
  measures "d34" diameter of A0
hole "Hole1" at (7.5, 15, 192.5) direction (0, -1, 0) diameter 6.78 depth 30 tip angle 118 countersink diameter 14.07 countersink angle 90
thread "Thread9" "ISO Metric profile 8.0 M8x1.25 6H"
hole "Hole2" at (332.5, 15, 192.5) direction (0, -1, 0) diameter 6.78 depth 30 tip angle 118 countersink diameter 14.07 countersink angle 90
thread "Thread10" "ISO Metric profile 8.0 M8x1.25 6H"
sketch "Sketch8" plane through (0, 15, 0) normal (0, 1, 0) x (-1, 0, 0)
  line L0 (-340, 200) -> (-223.097, 200)
  line L1 (-223.097, 200) -> (-223.097, 166.448)
  dimension "d45" = 116.903
  dimension "d46" = 33.552
  constraint horizontal L0
  constraint perpendicular L0 L1
  measures "d45" distance of L0.start L0.end
  measures "d46" distance of L0.end L1.end
hole "Hole3" at (223.097, 15, 166.448) direction (0, -1, 0) diameter 6.78 depth 30 tip angle 118 countersink diameter 14.07 countersink angle 90
thread "Thread11" "ISO Metric profile 8.0 M8x1.25 6H"
sketch "Sketch9" plane through (0, 15, 0) normal (0, 1, 0) x (-1, 0, 0)
  line L0 (-340, 0) -> (-223, 0)
  dimension "d52" = 117
  constraint horizontal L0
  measures "d52" distance of L0.start L0.end
sketch "Sketch10" plane through (0, 15, 0) normal (0, 1, 0) x (-1, 0, 0)
sketch "Sketch11" plane through (0, 0, 0) normal (0, -1, 0) x (1, 0, 0)
  circle A0 centre (223.097, 166.448) radius 3.3898
  circle A1 centre (332.5, 192.5) radius 3.3898
  circle A2 centre (7.5, 192.5) radius 3.3898
  circle A3 centre (272.5, 7.5) radius 3.3898
  circle A4 centre (7.5, 7.5) radius 3.3898
  circle A5 centre (67.5, 7.5) radius 3.3898
  circle A6 centre (332.5, 7.5) radius 3.3898
  line L0 (340, 200) -> (0, 200)
  line L1 (0, 200) -> (0, 0)
  line L2 (0, 0) -> (340, 0)
  line L3 (340, 0) -> (340, 200)
  line L4 (340, 0) -> (223.097, 0)
  line L5 (223.097, 0) -> (223.097, 20.528)
  dimension "d54" = 116.903
  dimension "d55" = 20.528
  constraint coincident L2.end L3.start
  constraint perpendicular L3 L4
  constraint perpendicular L2 L5
  measures "d54" distance of L2.end L4.end
  measures "d55" distance of L4.end L5.end
hole "Hole4" at (223.097, 0, 20.528) direction (0, 1, 0) diameter 6.78 depth 30 tip angle 118 countersink diameter 14.07 countersink angle 90
thread "Thread12" "ISO Metric profile 8.0 M8x1.25 6H"
sketch "Sketch12" plane through (0, 15, 0) normal (0, 1, 0) x (-1, 0, 0)
delete_face "DeleteFace5" 1 faces at (224.4138, 7.57, 163.3242)
delete_face "DeleteFace6" 1 faces at (217.6398, 13.8275, 164.3062)
sketch "Sketch13" plane through (0, 0, 0) normal (0, -1, 0) x (1, 0, 0)
  circle A0 centre (223.097, 20.528) radius 7.035
  circle A1 centre (332.5, 192.5) radius 3.3898
  circle A2 centre (7.5, 192.5) radius 3.3898
  circle A3 centre (272.5, 7.5) radius 3.3898
  circle A4 centre (7.5, 7.5) radius 3.3898
  circle A5 centre (67.5, 7.5) radius 3.3898
  circle A6 centre (332.5, 7.5) radius 3.3898
  line L0 (340, 200) -> (0, 200)
  line L1 (0, 200) -> (0, 0)
  line L2 (0, 0) -> (340, 0)
  line L3 (340, 0) -> (340, 200)
  line L4 (340, 200) -> (223.097, 200)
  line L5 (223.097, 200) -> (223.097, 165.92)
  dimension "d61" = 116.903
  dimension "d62" = 34.08
  constraint coincident L0.start L3.end
  constraint perpendicular L3 L4
  constraint perpendicular L0 L5
  measures "d61" distance of L0.start L4.end
  measures "d62" distance of L4.end L5.end
hole "Hole5" at (223.097, 0, 165.92) direction (0, 1, 0) diameter 6.78 depth 30 tip angle 118 countersink diameter 14.07 countersink angle 90
thread "Thread13" "ISO Metric profile 8.0 M8x1.25 6H"
sketch "Sketch14" plane through (0, 15, 0) normal (0, 1, 0) x (-1, 0, 0)
  circle A0 centre (-223.097, 165.92) radius 3.3898
  circle A1 centre (-223.097, 20.528) radius 3.3898
  circle A2 centre (-332.5, 192.5) radius 7.035
  circle A3 centre (-7.5, 192.5) radius 7.035
  circle A4 centre (-272.5, 7.5) radius 3.3898
  circle A5 centre (-7.5, 7.5) radius 3.3898
  circle A6 centre (-67.5, 7.5) radius 3.3898
  circle A7 centre (-332.5, 7.5) radius 3.3898
  line L0 (0, 200) -> (-340, 200)
  line L1 (-340, 200) -> (-340, 0)
  line L2 (-340, 0) -> (0, 0)
  line L3 (0, 0) -> (0, 200)
equation "d46 = 34.08 mm - 0.528 mm"
equation "d55 = 20 mm + 0.528 mm"
